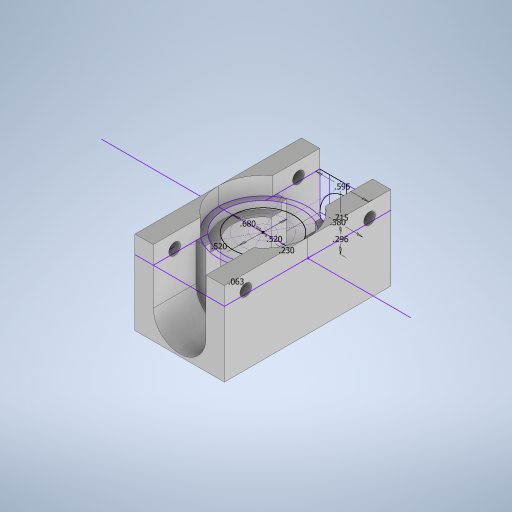
# Autodesk Inventor part: Ball Valve Mount 4
Saved by Autodesk Inventor 2024 (Build 280153000, 153)
## iProperties
Created: 2023-02-08
Part Number: Ball Valve Mount 4
Material: Generic
Document SubType Name: Modeling
Designer: tommy
Density: 1 g/cm^3
Appearance: Default
Author: tommy
Autodesk Inventor part; units mm, degrees
ref_plane "YZ Plane" through (0, 0, 0) normal (1, 0, 0) x (0, 1, 0)
ref_plane "XZ Plane" through (0, 0, 0) normal (0, 1, 0) x (-1, 0, 0)
ref_plane "XY Plane" through (0, 0, 0) normal (0, 0, 1) x (1, 0, 0)
sketch "Block1" plane through (0, 0, 0) normal (0, 0, 1) x (1, 0, 0)
  arc A0 (4.4042, -0.6007) -> (-4.4042, -0.6007) centre (0, 0) ccw
  arc A1 (-2.5167, -14.4402) -> (2.5167, -14.4402) centre (0, -14.097) ccw
  line L0 (-2.5167, -14.4402) -> (-4.4042, -0.6007)
  line L1 (4.4042, -0.6007) -> (2.5167, -14.4402)
  line L2 (-7.5501, -1.0297) -> (-5.6626, -14.8693)
  arc A2 (-5.6626, -14.8693) -> (5.6626, -14.8693) centre (0, -14.097) ccw
  line L3 (5.6626, -14.8693) -> (7.5501, -1.0297)
  arc A3 (7.5501, -1.0297) -> (-7.5501, -1.0297) centre (0, 0) ccw
  point P0 (0, -7.4025)
  dimension "d127" = 8.89
  dimension "d131" = 5.08
  dimension "d140" = 3.175
  measures "d127" diameter of A0
  measures "d131" diameter of A1
  measures "d140" distance between parallel lines of L0 L2
sketch "Sketch1" plane through (0, 0, 0) normal (0, 1, 0) x (-1, 0, 0)
  circle A0 centre (0, 0) radius 8.636
  line L0 (7.5565, 23.7871) -> (-7.5565, 23.7871)
  line L1 (7.5565, -23.7871) -> (-7.5565, -23.7871)
  line L2 (7.5565, 23.7871) -> (7.5565, 8.2342)
  line L3 (7.5565, -8.2342) -> (7.5565, -23.7871)
  arc A1 (7.5565, -8.2342) -> (7.5565, 8.2342) centre (0, 0) ccw
  arc A2 (-7.5565, 8.2342) -> (-7.5565, -8.2342) centre (0, 0) ccw
  line L4 (-7.5565, -23.7871) -> (-7.5565, -8.2342)
  line L5 (-7.5565, 8.2342) -> (-7.5565, 23.7871)
  line L6 (-9.144, -8.9047) -> (-9.144, -23.7871)
  line L7 (9.144, -23.7871) -> (9.144, -8.9047)
  line L8 (7.5565, -23.7871) -> (9.144, -23.7871)
  line L9 (9.144, -23.7871) -> (-9.144, -23.7871)
  line L10 (-7.5565, 23.7871) -> (-9.144, 23.7871)
  line L11 (-9.144, 23.7871) -> (9.144, 23.7871)
  circle A3 centre (0, 0) radius 11.176
  line L12 (46.1577, 0) -> (-42.2099, 0)
  circle A4 centre (0, 0) radius 2.921 construction
  circle A5 centre (0, 0) radius 6.604 construction
  circle A6 centre (0, 0) radius 6.604 construction
  line L13 (0, 0) -> (0, 23.3745) construction
  line L14 (-9.144, -18.796) -> (-7.5565, -18.796)
  line L15 (-9.144, -8.9047) -> (-9.144, -18.796)
  line L16 (-9.144, 23.7871) -> (-9.144, 8.9047)
  line L17 (9.144, -18.796) -> (9.144, -8.9047)
  line L18 (-12.7635, -23.7871) -> (12.7635, -23.7871)
  line L19 (12.7635, -23.7871) -> (12.7635, 23.7871)
  line L20 (12.7635, 23.7871) -> (-12.7635, 23.7871)
  line L21 (-12.7635, 23.7871) -> (-12.7635, -23.7871)
  line L22 (-12.7635, -23.7871) -> (12.7635, 23.7871) construction
  line L23 (12.7635, -23.7871) -> (-12.7635, 23.7871) construction
  circle A7 centre (0, 0) radius 12.7635
  point P0 (-7.5565, -8.2342)
  point P1 (-7.5565, 8.2342)
  point P2 (-8.636, 0)
  point P3 (8.636, 0)
  point P4 (-12.7635, 0)
  point P5 (-9.144, 21.9238)
  point P6 (11.176, 0)
  point P7 (-11.176, 0)
  point P8 (12.7635, 0)
  point P9 (-12.7635, 0)
  point P10 (-12.7635, 0)
  point P11 (-7.5565, -10.2862)
  point P12 (-7.5565, 10.2862)
  point P13 (12.7635, 0)
  point P14 (7.5565, -10.2862)
  point P15 (7.5565, 10.2862)
  dimension "d0" = 17.272
  dimension "d6" = 15.113
  dimension "d7" = 1.5875
  dimension "d31" = 5.842
  dimension "d32" = 13.208
  dimension "d49" = 13.208
  constraints: 48 end point, 7 centre point, 6 point on line, 5 coincident, 5 perpendicular, 4 point on circle, 3 vertical, 2 horizontal, 2 midpoint, 2 parallel, 1 collinear, 1 concentric, 3 other
  measures "d0" diameter of A0
  measures "d6" distance of L0.start L0.end
  measures "d7" distance between parallel lines of L4 L6
  measures "d31" diameter of A4
  measures "d32" diameter of A5
  measures "d49" diameter of A6
extrude "Extrusion1" add sketch "Sketch1" along normal blind 18.796 contours A0 L12 A2 A3 A1 | A1 L2 A7 L12 | L12 A7 L5 A2 | A3 L5 A7 L2 | A7 L2 L11 L20 L19 | L21 L20 L16 A7 | A7 L5 L0 L2 | A7 L16 L10 L5 picked at (-5.9238, 8.392)
extrude "Extrusion2" cut sketch "Sketch1" along normal blind 2.286 contours L12 A1 A3 A2 A0 | A0 L12 A2 A3 A1
sketch "Sketch2" plane through (-9.144, 0, 23.7871) normal (0, 0, 1) x (1, 0, 0)
  line L0 (9.144, 0) -> (9.144, 18.161)
  line L1 (9.144, 18.161) -> (9.144, 10.6426)
  circle A0 centre (9.144, 10.6426) radius 7.5184
  line L2 (16.6624, 10.6426) -> (16.6624, 0)
  line L3 (20.32, 0) -> (-2.032, 0) projected
  line L4 (1.6256, 10.6426) -> (1.6256, 0)
  line L5 (1.6256, 0) -> (16.6624, 0)
  circle A1 centre (9.144, 10.6426) radius 4.826
  line L6 (4.318, 10.6426) -> (4.318, 0)
  line L7 (13.97, 10.6426) -> (13.97, 0)
  line L8 (18.288, 0) -> (0, 0) projected
  line L9 (1.6256, 10.6426) -> (16.6624, 10.6426)
  point P0 (4.318, 0)
  point P1 (9.144, 7.5184)
  point P2 (4.318, 4.8775)
  point P3 (13.97, 4.8775)
  dimension "d12" = 18.161
  dimension "d13" = 7.5184
  dimension "d17" = 9.652
  constraints: 16 end point, 8 point on line, 5 point on circle, 3 perpendicular, 2 centre point, 2 coincident, 2 vertical, 1 horizontal, 1 parallel
  measures "d12" distance of L0.start L0.end
  measures "d13" distance of L0.end L1.end
  measures "d17" diameter of A1
extrude "Extrusion3" cut sketch "Sketch2" against normal blind 254 contours L3 L6 A0 L0 | L0 A0 L7 L3 | A0 L6 A1 L0 | L0 A1 L7 A0 | A1 L9 L0 | L0 L9 A1 | L9 A1 L0 | L0 A1 L9
extrude "Extrusion4" cut sketch "Sketch2" against normal blind 12.2174 contours A0 L6 A1 L0 | L0 A1 L7 A0 | L7 A0 L2 L3 | L3 L4 A0 L6 | A0 L9 L6 | L7 L9 A0 | L9 A0 L0 A1 | A1 L0 A0 L9
mirror "Mirror3" about plane through (12.7635, 0, 0) normal (0, 0, -1)
extrude "Extrusion21" add sketch "Sketch1" against normal blind 5.08 contours A7 L2 L11 L20 L19 | L19 L18 L7 A7 | A7 L6 L18 L21 | L21 L20 L16 A7 | A7 L7 L8 L3 | A7 L16 L10 L5 | L4 L14 L6 A7 | L4 L9 L6 L14
sketch "Sketch11" plane through (12.7635, 18.796, 23.7871) normal (1, 0, 0) x (0, 0, -1)
  line L0 (0, -0.635) -> (0, -15.6718) projected
  line L1 (47.5742, -18.796) -> (47.5742, -23.876) projected
  line L2 (47.5742, -19.7739) -> (0, -19.7739) construction
  line L3 (23.7871, -23.876) -> (0, -23.876) construction
  circle A0 centre (6.1087, -19.7739) radius 1.6637
  circle A1 centre (41.4655, -19.7739) radius 1.6637
  line L4 (13.5009, -18.796) -> (13.5009, -23.876) construction
  line L5 (12.2174, -8.1534) -> (12.2174, -18.796) construction
  line L6 (0, -23.876) -> (0, 0) construction
  line L7 (47.5742, 0) -> (47.5742, -23.876) construction
  point P0 (23.7871, -18.796)
  dimension "d145" = 4.1021
  dimension "d146" = 3.3274
  dimension "d147" = 3.3274
  dimension "d148" = 12.2174
  dimension "d150" = 6.1087
  dimension "d151" = 6.1087
  constraints: 3 point on line, 2 centre point, 2 end point, 1 perpendicular
  measures "d145" distance between parallel lines of L3 L2
  measures "d146" diameter of A0
  measures "d147" diameter of A1
  measures "d148" distance between parallel lines of L0 L5
  measures "d150" distance from line of L6 A0.centre
  measures "d151" distance from line of L7 A1.centre
extrude "Extrusion22" cut sketch "Sketch11" against normal blind 50.8
body "Solid1"
